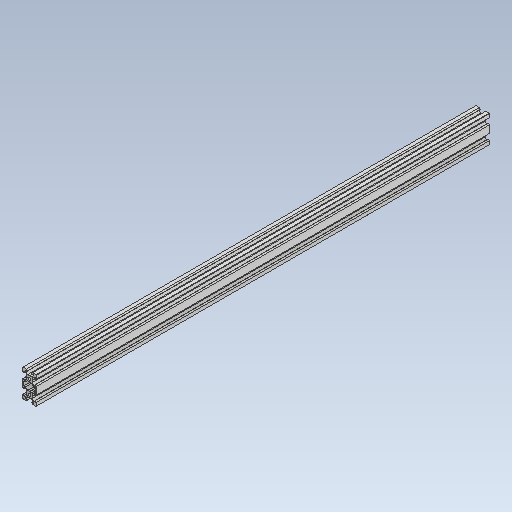
# Autodesk Inventor part: 0008-10-1019 V slot profiles
Saved by Autodesk Inventor 2020 (Build 240168000, 168)
## iProperties
Created: 2021-03-02
Part Number: 0008-10-1019 V slot profiles
Material: Generic
Document SubType Name: Modeling
Designer: Iulian Bors
Density: 1 g/cm^3
Appearance: Default
Description: Profil ALuminiu
Mass: 196.285 g
Surface Area: 1973.16 cm^2
Volume: 196.285 cm^3
Author: Iulian Bors
Subject: 1019
Autodesk Inventor part; units mm, degrees
ref_plane "YZ Plane" through (0, 0, 0) normal (1, 0, 0) x (0, 1, 0)
ref_plane "XZ Plane" through (0, 0, 0) normal (0, 1, 0) x (-1, 0, 0)
ref_plane "XY Plane" through (0, 0, 0) normal (0, 0, 1) x (1, 0, 0)
sketch "Sketch1" plane through (0, 0, 0) normal (0, 0, 1) x (1, 0, 0)
  line L0 (-0.5, 5.42) -> (-0.5, 0.5)
  arc A0 (-0.5, 0.5) -> (0, 0) centre (0, 0.5) ccw
  line L1 (0, 0) -> (4.92, 0)
  line L2 (4.92, 0) -> (6.375, 1.455)
  line L3 (6.375, 1.455) -> (6.375, 1.8)
  line L4 (6.375, 1.8) -> (4, 1.8)
  line L5 (4, 1.8) -> (4, 3.4393)
  line L6 (4, 3.4393) -> (6.6607, 6.1)
  line L7 (6.6607, 6.1) -> (9.3, 6.1)
  line L8 (9.3, 6.1) -> (9.5, 6.3)
  line L9 (9.5, 6.3) -> (9.7, 6.1)
  line L10 (9.7, 6.1) -> (12.3393, 6.1)
  line L11 (12.3393, 6.1) -> (15, 3.4393)
  line L12 (15, 3.4393) -> (15, 1.8)
  line L13 (15, 1.8) -> (12.625, 1.8)
  line L14 (12.625, 1.8) -> (12.625, 1.455)
  line L15 (12.625, 1.455) -> (14.08, 0)
  line L16 (14.08, 0) -> (19, 0)
  arc A1 (19, 0) -> (19.5, 0.5) centre (19, 0.5) ccw
  line L17 (19.5, 0.5) -> (19.5, 5.42)
  line L18 (19.5, 5.42) -> (18.045, 6.875)
  line L19 (18.045, 6.875) -> (17.7, 6.875)
  line L20 (17.7, 6.875) -> (17.7, 4.5)
  line L21 (17.7, 4.5) -> (16.0607, 4.5)
  line L22 (16.0607, 4.5) -> (13.4, 7.1607)
  line L23 (13.4, 7.1607) -> (13.4, 9.8)
  line L24 (13.4, 9.8) -> (13.2, 10)
  line L25 (13.2, 10) -> (13.4, 10.2)
  line L26 (13.4, 10.2) -> (13.4, 12.8393)
  line L27 (13.4, 12.8393) -> (16.0607, 15.5)
  line L28 (16.0607, 15.5) -> (17.7, 15.5)
  line L29 (17.7, 15.5) -> (17.7, 13.125)
  line L30 (17.7, 13.125) -> (18.045, 13.125)
  line L31 (18.045, 13.125) -> (19.5, 14.58)
  line L32 (19.5, 14.58) -> (19.5, 25.42)
  line L33 (19.5, 25.42) -> (18.045, 26.875)
  line L34 (18.045, 26.875) -> (17.7, 26.875)
  line L35 (17.7, 26.875) -> (17.7, 24.5)
  line L36 (17.7, 24.5) -> (16.0607, 24.5)
  line L37 (16.0607, 24.5) -> (13.4, 27.1607)
  line L38 (13.4, 27.1607) -> (13.4, 29.8)
  line L39 (13.4, 29.8) -> (13.2, 30)
  line L40 (13.2, 30) -> (13.4, 30.2)
  line L41 (13.4, 30.2) -> (13.4, 32.8393)
  line L42 (13.4, 32.8393) -> (16.0607, 35.5)
  line L43 (16.0607, 35.5) -> (17.7, 35.5)
  line L44 (17.7, 35.5) -> (17.7, 33.125)
  line L45 (17.7, 33.125) -> (18.045, 33.125)
  line L46 (18.045, 33.125) -> (19.5, 34.58)
  line L47 (19.5, 34.58) -> (19.5, 39.5)
  arc A2 (19.5, 39.5) -> (19, 40) centre (19, 39.5) ccw
  line L48 (19, 40) -> (14.08, 40)
  line L49 (14.08, 40) -> (12.625, 38.545)
  line L50 (12.625, 38.545) -> (12.625, 38.2)
  line L51 (12.625, 38.2) -> (15, 38.2)
  line L52 (15, 38.2) -> (15, 36.5607)
  line L53 (15, 36.5607) -> (12.3393, 33.9)
  line L54 (12.3393, 33.9) -> (9.7, 33.9)
  line L55 (9.7, 33.9) -> (9.5, 33.7)
  line L56 (9.5, 33.7) -> (9.3, 33.9)
  line L57 (9.3, 33.9) -> (6.6607, 33.9)
  line L58 (6.6607, 33.9) -> (4, 36.5607)
  line L59 (4, 36.5607) -> (4, 38.2)
  line L60 (4, 38.2) -> (6.375, 38.2)
  line L61 (6.375, 38.2) -> (6.375, 38.545)
  line L62 (6.375, 38.545) -> (4.92, 40)
  line L63 (4.92, 40) -> (0, 40)
  arc A3 (0, 40) -> (-0.5, 39.5) centre (0, 39.5) ccw
  line L64 (-0.5, 39.5) -> (-0.5, 34.58)
  line L65 (-0.5, 34.58) -> (0.955, 33.125)
  line L66 (0.955, 33.125) -> (1.3, 33.125)
  line L67 (1.3, 33.125) -> (1.3, 35.5)
  line L68 (1.3, 35.5) -> (2.9393, 35.5)
  line L69 (2.9393, 35.5) -> (5.6, 32.8393)
  line L70 (5.6, 32.8393) -> (5.6, 30.2)
  line L71 (5.6, 30.2) -> (5.8, 30)
  line L72 (5.8, 30) -> (5.6, 29.8)
  line L73 (5.6, 29.8) -> (5.6, 27.1607)
  line L74 (5.6, 27.1607) -> (2.9393, 24.5)
  line L75 (2.9393, 24.5) -> (1.3, 24.5)
  line L76 (1.3, 24.5) -> (1.3, 26.875)
  line L77 (1.3, 26.875) -> (0.955, 26.875)
  line L78 (0.955, 26.875) -> (-0.5, 25.42)
  line L79 (-0.5, 25.42) -> (-0.5, 14.58)
  line L80 (-0.5, 14.58) -> (0.955, 13.125)
  line L81 (0.955, 13.125) -> (1.3, 13.125)
  line L82 (1.3, 13.125) -> (1.3, 15.5)
  line L83 (1.3, 15.5) -> (2.9393, 15.5)
  line L84 (2.9393, 15.5) -> (5.6, 12.8393)
  line L85 (5.6, 12.8393) -> (5.6, 10.2)
  line L86 (5.6, 10.2) -> (5.8, 10)
  line L87 (5.8, 10) -> (5.6, 9.8)
  line L88 (5.6, 9.8) -> (5.6, 7.1607)
  line L89 (5.6, 7.1607) -> (2.9393, 4.5)
  line L90 (2.9393, 4.5) -> (1.3, 4.5)
  line L91 (1.3, 4.5) -> (1.3, 6.875)
  line L92 (1.3, 6.875) -> (0.955, 6.875)
  line L93 (0.955, 6.875) -> (-0.5, 5.42)
  line L94 (17.7, 23) -> (15.4393, 23)
  line L95 (17.7, 17) -> (17.7, 23)
  line L96 (15.4393, 17) -> (17.7, 17)
  line L97 (12.3393, 13.9) -> (15.4393, 17)
  line L98 (9.7, 13.9) -> (12.3393, 13.9)
  line L99 (9.5, 13.7) -> (9.7, 13.9)
  line L100 (9.3, 13.9) -> (9.5, 13.7)
  line L101 (6.6607, 13.9) -> (9.3, 13.9)
  line L102 (3.5607, 17) -> (6.6607, 13.9)
  line L103 (1.3, 17) -> (3.5607, 17)
  line L104 (1.3, 23) -> (1.3, 17)
  line L105 (3.5607, 23) -> (1.3, 23)
  line L106 (6.6607, 26.1) -> (3.5607, 23)
  line L107 (9.3, 26.1) -> (6.6607, 26.1)
  line L108 (9.5, 26.3) -> (9.3, 26.1)
  line L109 (9.7, 26.1) -> (9.5, 26.3)
  line L110 (12.3393, 26.1) -> (9.7, 26.1)
  line L111 (15.4393, 23) -> (12.3393, 26.1)
  circle A4 centre (9.5, 30) radius 2.1
  circle A5 centre (9.5, 10) radius 2.1
  point P0 (9.5, 20)
  constraints: 224 end point, 8 point on circle, 6 centre point
extrude "Extrusion1" add sketch "Sketch1" along normal mid plane 660
body "Solid1"
